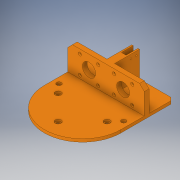
# Autodesk Inventor part: joint_1_base
Saved by Autodesk Inventor 2019 (Build 230136000, 136)
## iProperties
Created: 2019-12-25
Part Number: joint_1_base
Material: Пластик АБС
Document SubType Name: Modeling
Designer: Петров Иван
Density: 1.06 g/cm^3
Appearance: Оранжевый
Author: Петров Иван
Autodesk Inventor part; units mm, degrees
ref_plane "YZ Plane" through (0, 0, 0) normal (1, 0, 0) x (0, 1, 0)
ref_plane "XZ Plane" through (0, 0, 0) normal (0, 1, 0) x (-1, 0, 0)
ref_plane "XY Plane" through (0, 0, 0) normal (0, 0, 1) x (1, 0, 0)
sketch "Эскиз1" plane through (0, 0, 0) normal (0, 1, 0) x (-1, 0, 0)
  circle A0 centre (0, 41.5934) radius 3
  circle A1 centre (41.5934, 0) radius 3
  circle A2 centre (0, -41.5934) radius 3
  arc A3 (-20.609, 31.365) -> (-31.365, 20.609) centre (0, 0) ccw
  arc A4 (-45.7097, 6.2695) -> (-31.365, 20.609) centre (-73.1517, 48.0658) ccw
  arc A5 (-45.7097, 6.2695) -> (-45.7097, -6.2695) centre (-41.5934, 0) ccw
  arc A6 (-31.365, -20.609) -> (-45.7097, -6.2695) centre (-73.1517, -48.0658) ccw
  arc A7 (-31.365, -20.609) -> (-20.609, -31.365) centre (0, 0) ccw
  arc A8 (-6.2695, -45.7097) -> (-20.609, -31.365) centre (-48.0658, -73.1517) ccw
  arc A9 (-6.2695, -45.7097) -> (6.2695, -45.7097) centre (0, -41.5934) ccw
  arc A10 (20.609, -31.365) -> (6.2695, -45.7097) centre (48.0658, -73.1517) ccw
  arc A11 (20.609, -31.365) -> (31.365, -20.609) centre (0, 0) ccw
  arc A12 (45.7097, -6.2695) -> (31.365, -20.609) centre (73.1517, -48.0658) ccw
  arc A13 (45.7097, -6.2695) -> (45.7097, 6.2695) centre (41.5934, 0) ccw
  arc A14 (31.365, 20.609) -> (45.7097, 6.2695) centre (73.1517, 48.0658) ccw
  arc A15 (31.365, 20.609) -> (20.609, 31.365) centre (0, 0) ccw
  arc A16 (6.2695, 45.7097) -> (20.609, 31.365) centre (48.0658, 73.1517) ccw
  arc A17 (6.2695, 45.7097) -> (-6.2695, 45.7097) centre (0, 41.5934) ccw
  arc A18 (-20.609, 31.365) -> (-6.2695, 45.7097) centre (-48.0658, 73.1517) ccw
  circle A19 centre (-41.5934, 0) radius 3
  circle A20 centre (41.5934, 0) radius 3
  circle A21 centre (0, 41.5934) radius 3
  circle A22 centre (-41.5934, 0) radius 3
  circle A23 centre (0, -41.5934) radius 3
  circle A24 centre (0, 0) radius 65
  constraints: 32 point on circle, 25 centre point
extrude "Выдавливание1" add sketch "Эскиз1" along normal blind 5 contours A18 A17 A16 A15 A14 A13 A12 A11 A10 A9 A8 A7 A6 A5 A4 A3 | A24
sketch "Эскиз2" plane through (0, 5, 0) normal (0, 1, 0) x (1, 0, 0)
  circle A0 centre (0, 0) radius 65 projected
  line L0 (65, 0) -> (65, 90)
  line L1 (65, 90) -> (-65, 90)
  line L2 (-65, 90) -> (-65, 0)
  circle A1 centre (41.5934, 0) radius 3 projected
  circle A2 centre (41.5934, 0) radius 3
  circle A3 centre (-41.5934, 0) radius 3 projected
  circle A4 centre (-41.5934, 0) radius 3
  line L3 (-65, 0) -> (-44.5934, 0)
  line L4 (-38.5934, 0) -> (38.5934, 0)
  line L5 (44.5934, 0) -> (65, 0)
  dimension "d2" = 90
  constraints: 12 end point, 4 parallel, 4 point on circle, 3 horizontal, 3 perpendicular, 2 centre point, 2 coincident, 1 concentric, 1 horizontal alignment, 1 other
  measures "d2" distance of L0.end L0.start
extrude "Выдавливание2" add sketch "Эскиз2" against normal blind 5 contours L5 A1 L4 A3 L3 A0 | A0 L2 L1 L0 picked at (0, 22.5961)
chamfer "Фаска1" distance 5 angle 45 2 edges at (65, 2.5, -90) (-65, 2.5, -90)
sketch "Эскиз3" plane through (0, 5, 0) normal (0, 1, 0) x (1, 0, 0)
  line L0 (60, 90) -> (-60, 90)
  line L1 (-8, 80.5) -> (-8, 90)
  line L2 (-40, 47.8) -> (-18, 47.8)
  line L3 (-50, 49.8) -> (-50, 57.5)
  line L4 (-50, 80.5) -> (-50, 90)
  line L5 (-8, 49.8) -> (-8, 57.5)
  line L6 (8, 49.8) -> (8, 57.5)
  line L7 (8, 80.5) -> (8, 90)
  line L8 (50, 49.8) -> (50, 57.5)
  line L9 (50, 80.5) -> (50, 90)
  line L10 (18, 47.8) -> (40, 47.8)
  line L11 (-8, 47.8) -> (-50, 47.8)
  line L12 (-50, 47.8) -> (-50, 90)
  line L13 (-50, 90) -> (-8, 90)
  line L14 (-8, 90) -> (-8, 47.8)
  line L15 (8, 90) -> (50, 90)
  line L16 (50, 90) -> (50, 47.8)
  line L17 (50, 47.8) -> (8, 47.8)
  line L18 (8, 47.8) -> (8, 90)
  line L19 (-65, 0) -> (-65, 85) projected
  line L20 (65, 85) -> (65, 0) projected
  line L21 (-65, 47.8) -> (65, 47.8)
  line L22 (65, 47.8) -> (65, 39.8)
  line L23 (65, 39.8) -> (-65, 39.8)
  line L24 (-65, 39.8) -> (-65, 47.8)
  point P0 (0, 0)
  dimension "d8" = 8
  constraints: 46 end point, 6 parallel, 3 horizontal, 3 perpendicular, 3 point on line
  measures "d8" distance of L21.end L22.end
extrude "Выдавливание3" add sketch "Эскиз3" against normal blind 49 contours L21 L20 L23 L19 L11 L2 L17 L10
sketch "Эскиз5" plane through (-65, 0, -39.8) normal (0, 0, 1) x (1, 0, 0)
  circle A0 centre (94, -21) radius 11.3
  circle A1 centre (36, -21) radius 11
  line L0 (130, 0) -> (130, -44)
  line L1 (130, -44) -> (0, -44)
  point P0 (65, 0)
  dimension "d15" = 22.6
  constraints: 4 end point, 2 centre point
  measures "d15" diameter of A0
extrude "Выдавливание4" cut sketch "Эскиз5" against normal blind 44
sketch "Эскиз6" plane through (-65, 0, -39.8) normal (0, 0, 1) x (1, 0, 0)
  line L0 (111.5, -42) -> (115, -38.5)
  line L1 (115, -38.5) -> (115, -3.5)
  line L2 (115, -3.5) -> (111.5, 0)
  line L3 (111.5, 0) -> (76.5, 0)
  line L4 (76.5, 0) -> (73, -3.5)
  line L5 (73, -3.5) -> (73, -38.5)
  line L6 (73, -38.5) -> (76.5, -42)
  line L7 (76.5, -42) -> (111.5, -42)
  circle A0 centre (94, -21) radius 11.3
  circle A1 centre (109.5, -5.5) radius 1.25
  circle A2 centre (78.5, -5.5) radius 1.25
  circle A3 centre (78.5, -36.5) radius 1.25
  circle A4 centre (109.5, -36.5) radius 1.25
  line L8 (86, -48) -> (88, -48)
  line L9 (88, -41.8) -> (88, -48)
  line L10 (80.5828, -41.8) -> (88, -41.8)
  line L11 (73.2, -34.4172) -> (80.5828, -41.8)
  line L12 (73.2, -7.5828) -> (73.2, -34.4172)
  line L13 (80.5828, -0.2) -> (73.2, -7.5828)
  line L14 (107.4172, -0.2) -> (80.5828, -0.2)
  line L15 (114.8, -7.5828) -> (107.4172, -0.2)
  line L16 (114.8, -34.4172) -> (114.8, -7.5828)
  line L17 (107.4172, -41.8) -> (114.8, -34.4172)
  line L18 (100, -41.8) -> (107.4172, -41.8)
  line L19 (100, -41.8) -> (100, -48)
  line L20 (100, -48) -> (102, -48)
  line L21 (102, -48) -> (102, -42)
  line L22 (102, -42) -> (111.5, -42)
  line L23 (111.5, -42) -> (115, -38.5)
  line L24 (115, -38.5) -> (115, -3.5)
  line L25 (115, -3.5) -> (111.5, 0)
  line L26 (111.5, 0) -> (76.5, 0)
  line L27 (76.5, 0) -> (73, -3.5)
  line L28 (73, -3.5) -> (73, -38.5)
  line L29 (73, -38.5) -> (76.5, -42)
  line L30 (76.5, -42) -> (86, -42)
  line L31 (86, -42) -> (86, -48)
  circle A5 centre (94, -21) radius 11.3 projected
  circle A6 centre (36, -21) radius 11 projected
  line L32 (53.5, -42) -> (57, -38.5)
  line L33 (57, -38.5) -> (57, -3.5)
  line L34 (57, -3.5) -> (53.5, 0)
  line L35 (53.5, 0) -> (18.5, 0)
  line L36 (18.5, 0) -> (15, -3.5)
  line L37 (15, -3.5) -> (15, -38.5)
  line L38 (15, -38.5) -> (18.5, -42)
  line L39 (18.5, -42) -> (53.5, -42)
  circle A7 centre (36, -21) radius 11.3
  circle A8 centre (51.5, -5.5) radius 1.25
  circle A9 centre (20.5, -5.5) radius 1.25
  circle A10 centre (20.5, -36.5) radius 1.25
  circle A11 centre (51.5, -36.5) radius 1.25
  line L40 (28, -48) -> (30, -48)
  line L41 (30, -41.8) -> (30, -48)
  line L42 (22.5828, -41.8) -> (30, -41.8)
  line L43 (15.2, -34.4172) -> (22.5828, -41.8)
  line L44 (15.2, -7.5828) -> (15.2, -34.4172)
  line L45 (22.5828, -0.2) -> (15.2, -7.5828)
  line L46 (49.4172, -0.2) -> (22.5828, -0.2)
  line L47 (56.8, -7.5828) -> (49.4172, -0.2)
  line L48 (56.8, -34.4172) -> (56.8, -7.5828)
  line L49 (49.4172, -41.8) -> (56.8, -34.4172)
  line L50 (42, -41.8) -> (49.4172, -41.8)
  line L51 (42, -41.8) -> (42, -48)
  line L52 (42, -48) -> (44, -48)
  line L53 (44, -48) -> (44, -42)
  line L54 (44, -42) -> (53.5, -42)
  line L55 (53.5, -42) -> (57, -38.5)
  line L56 (57, -38.5) -> (57, -3.5)
  line L57 (57, -3.5) -> (53.5, 0)
  line L58 (53.5, 0) -> (18.5, 0)
  line L59 (18.5, 0) -> (15, -3.5)
  line L60 (15, -3.5) -> (15, -38.5)
  line L61 (15, -38.5) -> (18.5, -42)
  line L62 (18.5, -42) -> (28, -42)
  line L63 (28, -42) -> (28, -48)
  point P0 (65, 0)
  constraints: 128 end point, 10 centre point
extrude "Выдавливание5" cut sketch "Эскиз6" against normal blind 44 contours A1 | A2 | A3 | A4 | A8 | A9 | A10 | A11
chamfer "Фаска3" distance 8 angle 45 2 edges at (65, -44, -43.8) (-65, -44, -43.8)
sketch "Эскиз7" plane through (0, 0, 0) normal (0, -1, 0) x (1, 0, 0)
  circle A0 centre (0, 41.5934) radius 3 projected
  circle A1 centre (0, 41.5934) radius 5
  circle A2 centre (-41.5934, 0) radius 3 projected
  circle A3 centre (-41.5934, 0) radius 5
  circle A4 centre (41.5934, 0) radius 3 projected
  circle A5 centre (41.5934, 0) radius 5
  point P0 (0, 0)
  dimension "d22" = 10
  dimension "d23" = 10
  dimension "d24" = 10
  constraints: 3 centre point, 3 coincident
  measures "d22" diameter of A1
  measures "d23" diameter of A3
  measures "d24" diameter of A5
extrude "Выдавливание6" cut sketch "Эскиз7" against normal blind 3 contours A1 | A2 | A3 | A5
chamfer "Фаска4" distance 1.5 angle 45 8 edges at (43.25, -36.5, -39.8) (12.25, -36.5, -39.8) (12.25, -5.5, -39.8) (43.25, -5.5, -39.8) (-14.75, -36.5, -39.8) (-14.75, -5.5, -39.8) (-45.75, -5.5, -39.8) (-45.75, -36.5, -39.8)
sketch "Эскиз8" plane through (0, 5, 0) normal (0, 1, 0) x (1, 0, 0)
  circle A0 centre (-55, 14.8) radius 4
  circle A1 centre (55, 14.8) radius 4
  line L0 (60, 90) -> (-60, 90)
  point P0 (0, 0)
  constraints: 2 centre point, 2 end point
extrude "Выдавливание7" cut sketch "Эскиз8" against normal through all
sketch "Эскиз9" plane through (65, 0, -47.8) normal (0, 0, -1) x (-1, 0, 0)
  line L0 (122, -44) -> (8, -44) projected
  line L1 (65, -44) -> (65, -22)
  line L2 (71.5, 0) -> (58.5, 0)
  line L3 (58.5, 0) -> (58.5, -44)
  line L4 (58.5, -44) -> (71.5, -44)
  line L5 (71.5, -44) -> (71.5, 0)
  line L6 (71.5, 0) -> (58.5, -44) construction
  line L7 (58.5, 0) -> (71.5, -44) construction
  point P0 (65, 0)
  dimension "d32" = 13
  dimension "d34" = 22
  constraints: 14 end point, 3 midpoint, 2 parallel, 1 horizontal, 1 perpendicular, 1 point on line, 1 vertical
  measures "d32" distance of L4.end L3.end
  measures "d34" distance of L1.start L1.end
extrude "Выдавливание8" add sketch "Эскиз9" along normal up to surface (42.2 mm away)
sketch "Эскиз10" plane through (0, -44, 0) normal (0, -1, 0) x (1, 0, 0)
  line L0 (-6.5, -90) -> (6.5, -90) projected
  line L1 (0, -90) -> (0, -79.9)
  line L2 (-4, -90) -> (4, -90)
  line L3 (4, -90) -> (4, -69.8)
  line L4 (4, -69.8) -> (-4, -69.8)
  line L5 (-4, -69.8) -> (-4, -90)
  line L6 (-4, -90) -> (4, -69.8) construction
  line L7 (4, -90) -> (-4, -69.8) construction
  line L8 (-57, -47.8) -> (-57, -39.8) projected
  line L9 (-57, -47.8) -> (-6.5, -47.8) projected
  line L10 (-6.5, -47.8) -> (-6.5, -90) projected
  line L11 (-6.5, -90) -> (6.5, -90) projected
  line L12 (6.5, -47.8) -> (6.5, -90) projected
  line L13 (6.5, -47.8) -> (57, -47.8) projected
  line L14 (57, -39.8) -> (57, -47.8) projected
  line L15 (57, -39.8) -> (-57, -39.8) projected
  line L16 (-6.5, -47.8) -> (-6.5, -90) projected
  line L17 (-6.5, -47.8) -> (6.5, -47.8)
  line L18 (6.5, -47.8) -> (6.5, -90)
  line L19 (4, -90) -> (6.5, -90)
  line L20 (-4, -90) -> (-6.5, -90)
  line L21 (-6.5, -90) -> (-6.5, -47.8)
  point P0 (0, 0)
  dimension "d37" = 10.1
  dimension "d38" = 8
  dimension "d39" = 20.2
  constraints: 24 end point, 3 equal length, 3 midpoint, 3 perpendicular, 1 horizontal, 1 vertical
  measures "d37" distance of L1.start L1.end
  measures "d38" distance of L4.end L3.end
  measures "d39" distance of L3.end L2.end
extrude "Выдавливание9" cut sketch "Эскиз10" against normal blind 18 contours L5 L4 L3 L0
sketch "Эскиз11" plane through (-6.5, -44, -47.8) normal (-1, 0, 0) x (0, 0, 1)
  line L0 (-42.2, 18) -> (-22, 18) projected
  line L1 (-22, 0) -> (-22, 18) projected
  arc A0 (-42.133, -0.5583) -> (-42.033, -0.4583) centre (-42.133, -0.4583) ccw
  line L2 (-42.033, -0.4583) -> (-42.033, 8.6917)
  arc A1 (-42.033, 8.6917) -> (-42.133, 8.7917) centre (-42.133, 8.6917) ccw
  line L3 (-22.333, -1.0583) -> (-22.8455, -1.0583)
  line L4 (-22.8455, -1.0583) -> (-22.9372, 0.3757)
  arc A2 (-22.9372, 0.3757) -> (-27.1287, 0.3757) centre (-25.033, 0.2417) ccw
  line L5 (-27.1287, 0.3757) -> (-27.2204, -1.0583)
  line L6 (-27.2204, -1.0583) -> (-31.5087, -1.0583)
  arc A3 (-31.5794, -1.029) -> (-31.5087, -1.0583) centre (-31.5087, -0.9583) ccw
  line L7 (-31.5794, -1.029) -> (-31.9037, -0.7048)
  arc A4 (-31.9037, -0.7048) -> (-32.2572, -0.5583) centre (-32.2572, -1.0583) ccw
  line L8 (-32.2572, -0.5583) -> (-41.933, -0.5583)
  arc A5 (-42.033, -0.4583) -> (-41.933, -0.5583) centre (-41.933, -0.4583) ccw
  arc A6 (-41.933, 8.7917) -> (-42.033, 8.6917) centre (-41.933, 8.6917) ccw
  line L9 (-41.933, 8.7917) -> (-39.0072, 8.7917)
  arc A7 (-39.0072, 8.7917) -> (-38.6537, 8.9381) centre (-39.0072, 9.2917) ccw
  line L10 (-38.6537, 8.9381) -> (-38.3294, 9.2624)
  arc A8 (-38.2587, 9.2917) -> (-38.3294, 9.2624) centre (-38.2587, 9.1917) ccw
  line L11 (-38.2587, 9.2917) -> (-35.5072, 9.2917)
  arc A9 (-35.4365, 9.2624) -> (-35.5072, 9.2917) centre (-35.5072, 9.1917) ccw
  line L12 (-35.4365, 9.2624) -> (-35.1122, 8.9381)
  arc A10 (-35.1122, 8.9381) -> (-34.7587, 8.7917) centre (-34.7587, 9.2917) ccw
  line L13 (-34.7587, 8.7917) -> (-29.5072, 8.7917)
  arc A11 (-29.5072, 8.7917) -> (-29.1537, 8.9381) centre (-29.5072, 9.2917) ccw
  line L14 (-29.1537, 8.9381) -> (-28.8294, 9.2624)
  arc A12 (-28.7587, 9.2917) -> (-28.8294, 9.2624) centre (-28.7587, 9.1917) ccw
  line L15 (-28.7587, 9.2917) -> (-26.0072, 9.2917)
  arc A13 (-25.9365, 9.2624) -> (-26.0072, 9.2917) centre (-26.0072, 9.1917) ccw
  line L16 (-25.9365, 9.2624) -> (-25.6122, 8.9381)
  arc A14 (-25.6122, 8.9381) -> (-25.2587, 8.7917) centre (-25.2587, 9.2917) ccw
  line L17 (-25.2587, 8.7917) -> (-22.333, 8.7917)
  arc A15 (-22.233, 8.6917) -> (-22.333, 8.7917) centre (-22.333, 8.6917) ccw
  line L18 (-22.233, 8.6917) -> (-22.233, -0.9583)
  arc A16 (-22.333, -1.0583) -> (-22.233, -0.9583) centre (-22.333, -0.9583) ccw
  circle A17 centre (-27.383, 6.7417) radius 1.25
  circle A18 centre (-36.883, 6.7417) radius 1.25
  line L19 (-38.0563, 4.4917) -> (-37.4396, 3.1917)
  line L20 (-37.4396, 3.1917) -> (-37.423, 3.1917)
  line L21 (-37.423, 3.1917) -> (-36.823, 4.4917)
  line L22 (-36.823, 4.4917) -> (-36.9498, 4.4917)
  line L23 (-36.9498, 4.4917) -> (-37.142, 4.075)
  line L24 (-37.142, 4.075) -> (-37.7313, 4.075)
  line L25 (-37.7313, 4.075) -> (-37.9289, 4.4917)
  line L26 (-37.9289, 4.4917) -> (-38.0563, 4.4917)
  spline S0 degree 3 poles (-35.2363, 3.5552) (-35.2365, 3.5463) (-35.237, 3.5289) (-35.2411, 3.5032) (-35.2473, 3.4785) (-35.2562, 3.4546) (-35.2679, 3.4318) (-35.2822, 3.41) (-35.2987, 3.389) (-35.3178, 3.3692) (-35.3387, 3.3511) (-35.3609, 3.3351) (-35.3843, 3.3217) (-35.4089, 3.3108) (-35.4346, 3.3022) (-35.4615, 3.2962) (-35.4895, 3.2924) (-35.5086, 3.2919) (-35.5183, 3.2917) knots 0 0 0 0 0.061965 0.122122 0.180988 0.239933 0.299906 0.359989 0.421776 0.486576 0.551535 0.615018 0.677259 0.73973 0.80305 0.866495 0.931973 1 1 1 1
  spline S1 degree 3 poles (-35.5183, 3.2917) (-35.5285, 3.2919) (-35.5485, 3.2925) (-35.5778, 3.2961) (-35.6057, 3.3024) (-35.6324, 3.311) (-35.6579, 3.322) (-35.682, 3.3356) (-35.7046, 3.3518) (-35.7259, 3.3703) (-35.7456, 3.3908) (-35.7628, 3.4137) (-35.7779, 3.4385) (-35.7911, 3.4652) (-35.8017, 3.494) (-35.8099, 3.5248) (-35.8164, 3.5575) (-35.8185, 3.5801) (-35.8196, 3.5917) knots 0 0 0 0 0.064439 0.126547 0.186887 0.245878 0.304041 0.362191 0.420976 0.48066 0.5406 0.600689 0.661936 0.724443 0.789038 0.856314 0.926352 1 1 1 1
  line L27 (-35.8196, 3.5917) -> (-35.9363, 3.5917)
  spline S2 degree 3 poles (-35.9363, 3.5917) (-35.9355, 3.5762) (-35.934, 3.5458) (-35.927, 3.5015) (-35.917, 3.4591) (-35.9029, 3.4191) (-35.8853, 3.3809) (-35.8642, 3.3449) (-35.8393, 3.3111) (-35.811, 3.2799) (-35.7802, 3.2512) (-35.7471, 3.2264) (-35.7122, 3.2055) (-35.6758, 3.188) (-35.6373, 3.1749) (-35.5973, 3.1652) (-35.5554, 3.1593) (-35.5268, 3.1587) (-35.5123, 3.1583) knots 0 0 0 0 0.068791 0.135103 0.198979 0.261904 0.323495 0.385195 0.446969 0.509765 0.572251 0.633405 0.693251 0.752583 0.812579 0.873275 0.93555 1 1 1 1
  spline S3 degree 3 poles (-35.5123, 3.1583) (-35.4981, 3.1587) (-35.4701, 3.1593) (-35.4292, 3.165) (-35.3903, 3.1738) (-35.3534, 3.1862) (-35.3188, 3.2028) (-35.2864, 3.2228) (-35.2556, 3.2459) (-35.2279, 3.2731) (-35.2024, 3.3021) (-35.1805, 3.3331) (-35.1617, 3.3652) (-35.146, 3.3985) (-35.1345, 3.4333) (-35.1257, 3.4693) (-35.1208, 3.5066) (-35.12, 3.5319) (-35.1196, 3.5448) knots 0 0 0 0 0.069475 0.136517 0.200789 0.26383 0.325735 0.387291 0.449509 0.512968 0.576275 0.63758 0.697903 0.757172 0.816599 0.876653 0.93729 1 1 1 1
  spline S4 degree 3 poles (-35.1196, 3.5448) (-35.1203, 3.5629) (-35.1215, 3.5988) (-35.1322, 3.6516) (-35.1488, 3.7027) (-35.1689, 3.7438) (-35.1891, 3.7769) (-35.2073, 3.8042) (-35.2287, 3.8336) (-35.2535, 3.865) (-35.2811, 3.8986) (-35.312, 3.9344) (-35.3462, 3.9721) (-35.3702, 3.9979) (-35.3826, 4.0112) knots 0 0 0 0 0.098702 0.195672 0.292422 0.391343 0.444462 0.504229 0.570352 0.642546 0.722288 0.807921 0.90047 1 1 1 1
  line L28 (-35.3826, 4.0112) -> (-35.7079, 4.3583)
  line L29 (-35.7079, 4.3583) -> (-35.103, 4.3583)
  line L30 (-35.103, 4.3583) -> (-35.103, 4.4917)
  line L31 (-35.103, 4.4917) -> (-35.9863, 4.4917)
  line L32 (-35.9863, 4.4917) -> (-35.4821, 3.9537)
  spline S5 degree 3 poles (-35.4821, 3.9537) (-35.4699, 3.9408) (-35.4463, 3.9162) (-35.4129, 3.8803) (-35.383, 3.847) (-35.3562, 3.8163) (-35.3333, 3.7878) (-35.3129, 3.7625) (-35.2965, 3.7392) (-35.2788, 3.7122) (-35.2617, 3.6792) (-35.2469, 3.6389) (-35.2379, 3.5974) (-35.2368, 3.5693) (-35.2363, 3.5552) knots 0 0 0 0 0.110803 0.212829 0.306101 0.390647 0.466924 0.534481 0.593587 0.644557 0.7362 0.825024 0.911986 1 1 1 1
  line L33 (-34.7263, 3.8417) -> (-34.593, 3.1917)
  line L34 (-34.593, 3.1917) -> (-34.0596, 3.1917)
  line L35 (-34.0596, 3.1917) -> (-34.0596, 3.325)
  line L36 (-34.0596, 3.325) -> (-34.5018, 3.325)
  line L37 (-34.5018, 3.325) -> (-34.5719, 3.6669)
  spline S6 degree 3 poles (-34.5719, 3.6669) (-34.5581, 3.6631) (-34.5314, 3.6558) (-34.4921, 3.6476) (-34.4547, 3.6427) (-34.4305, 3.642) (-34.4187, 3.6417) knots 0 0 0 0 0.275068 0.532901 0.773973 1 1 1 1
  spline S7 degree 3 poles (-34.4187, 3.6417) (-34.4042, 3.642) (-34.3757, 3.6426) (-34.3339, 3.6485) (-34.294, 3.6579) (-34.2562, 3.6709) (-34.2202, 3.6876) (-34.1865, 3.7084) (-34.1544, 3.7328) (-34.1248, 3.7608) (-34.0978, 3.7916) (-34.0741, 3.8247) (-34.054, 3.8598) (-34.0378, 3.8972) (-34.0249, 3.9366) (-34.0163, 3.9783) (-34.0106, 4.0219) (-34.01, 4.0517) (-34.0096, 4.0669) knots 0 0 0 0 0.065808 0.129394 0.190894 0.251281 0.310815 0.370371 0.430768 0.492881 0.555104 0.616067 0.677256 0.73826 0.800762 0.864778 0.931045 1 1 1 1
  spline S8 degree 3 poles (-34.0096, 4.0669) (-34.0099, 4.0775) (-34.0104, 4.0986) (-34.0129, 4.1298) (-34.0177, 4.1604) (-34.0241, 4.1904) (-34.0325, 4.2196) (-34.0426, 4.2482) (-34.055, 4.2759) (-34.0686, 4.3032) (-34.084, 4.3293) (-34.101, 4.3536) (-34.1189, 4.3767) (-34.1383, 4.3982) (-34.1591, 4.418) (-34.1813, 4.4361) (-34.2046, 4.453) (-34.2293, 4.468) (-34.255, 4.4817) (-34.282, 4.4929) (-34.3096, 4.503) (-34.3384, 4.511) (-34.3681, 4.5173) (-34.3989, 4.5216) (-34.4307, 4.5247) (-34.4522, 4.5249) (-34.463, 4.525) knots 0 0 0 0 0.044014 0.087434 0.130118 0.172554 0.214555 0.256298 0.298438 0.340849 0.382715 0.423924 0.464246 0.504074 0.543862 0.583567 0.623094 0.663229 0.703551 0.743938 0.784541 0.82575 0.867757 0.910745 0.954914 1 1 1 1
  spline S9 degree 3 poles (-34.463, 4.525) (-34.476, 4.5248) (-34.5014, 4.5242) (-34.5388, 4.519) (-34.5747, 4.5114) (-34.6089, 4.5) (-34.6418, 4.4858) (-34.6727, 4.4677) (-34.7027, 4.4473) (-34.7304, 4.4232) (-34.756, 4.3969) (-34.779, 4.3683) (-34.7995, 4.3379) (-34.8171, 4.3057) (-34.8322, 4.2716) (-34.844, 4.2355) (-34.8535, 4.1976) (-34.8576, 4.1716) (-34.8596, 4.1583) knots 0 0 0 0 0.065421 0.128708 0.190236 0.250724 0.310637 0.370766 0.431615 0.493523 0.555883 0.617342 0.678668 0.740711 0.802985 0.866803 0.932347 1 1 1 1
  line L38 (-34.8596, 4.1583) -> (-34.743, 4.1583)
  spline S10 degree 3 poles (-34.743, 4.1583) (-34.7401, 4.1707) (-34.7346, 4.1946) (-34.7225, 4.228) (-34.7077, 4.2579) (-34.69, 4.2845) (-34.669, 4.3076) (-34.6451, 4.3283) (-34.6182, 4.3469) (-34.5883, 4.3625) (-34.5568, 4.3757) (-34.5239, 4.3845) (-34.4903, 4.3907) (-34.4676, 4.3914) (-34.4562, 4.3917) knots 0 0 0 0 0.094687 0.181994 0.264377 0.34218 0.418618 0.496509 0.577369 0.661511 0.746733 0.831258 0.915206 1 1 1 1
  spline S11 degree 3 poles (-34.4562, 4.3917) (-34.4451, 4.3914) (-34.4232, 4.3908) (-34.391, 4.3862) (-34.3598, 4.379) (-34.3301, 4.3684) (-34.3013, 4.3554) (-34.2741, 4.3388) (-34.2478, 4.3197) (-34.2231, 4.2978) (-34.2005, 4.2737) (-34.1806, 4.2479) (-34.1639, 4.2204) (-34.1499, 4.1916) (-34.1393, 4.1612) (-34.1317, 4.1295) (-34.1272, 4.0962) (-34.1266, 4.0735) (-34.1263, 4.062) knots 0 0 0 0 0.064207 0.126425 0.18768 0.248216 0.308305 0.369661 0.431699 0.495947 0.559758 0.622295 0.683911 0.745092 0.80674 0.869087 0.93329 1 1 1 1
  spline S12 degree 3 poles (-34.1263, 4.062) (-34.1265, 4.0516) (-34.127, 4.0311) (-34.1309, 4.0013) (-34.1377, 3.973) (-34.1472, 3.9462) (-34.1592, 3.9209) (-34.1738, 3.897) (-34.1914, 3.8748) (-34.2115, 3.8543) (-34.2335, 3.8354) (-34.2578, 3.8193) (-34.2839, 3.8058) (-34.3115, 3.7941) (-34.3412, 3.7857) (-34.3724, 3.7794) (-34.4055, 3.7758) (-34.4282, 3.7753) (-34.4398, 3.775) knots 0 0 0 0 0.065351 0.127916 0.18836 0.247216 0.30563 0.36377 0.422661 0.482687 0.5433 0.604118 0.664965 0.727413 0.791468 0.858055 0.927037 1 1 1 1
  spline S13 degree 3 poles (-34.4398, 3.775) (-34.4499, 3.7752) (-34.4707, 3.7757) (-34.5026, 3.7789) (-34.5362, 3.7842) (-34.5712, 3.7915) (-34.6078, 3.801) (-34.646, 3.8124) (-34.6857, 3.8261) (-34.7125, 3.8364) (-34.7263, 3.8417) knots 0 0 0 0 0.102203 0.211023 0.3251 0.446502 0.573788 0.708901 0.850358 1 1 1 1
  line L39 (-31.2796, 4.4917) -> (-30.663, 3.1917)
  line L40 (-30.663, 3.1917) -> (-30.6463, 3.1917)
  line L41 (-30.6463, 3.1917) -> (-30.0463, 4.4917)
  line L42 (-30.0463, 4.4917) -> (-30.1731, 4.4917)
  line L43 (-30.1731, 4.4917) -> (-30.3653, 4.075)
  line L44 (-30.3653, 4.075) -> (-30.9546, 4.075)
  line L45 (-30.9546, 4.075) -> (-31.1523, 4.4917)
  line L46 (-31.1523, 4.4917) -> (-31.2796, 4.4917)
  spline S14 degree 3 poles (-29.7696, 3.8341) (-29.769, 3.8107) (-29.7679, 3.7647) (-29.7583, 3.6972) (-29.7427, 3.6325) (-29.7207, 3.5708) (-29.6927, 3.5117) (-29.6581, 3.4557) (-29.6174, 3.4024) (-29.5708, 3.3526) (-29.5197, 3.3071) (-29.465, 3.267) (-29.4068, 3.2337) (-29.3457, 3.2058) (-29.2812, 3.1844) (-29.2136, 3.1695) (-29.1429, 3.1601) (-29.0947, 3.1589) (-29.0701, 3.1583) knots 0 0 0 0 0.064558 0.127014 0.187955 0.248014 0.307748 0.368235 0.42947 0.492743 0.556258 0.618217 0.679655 0.741246 0.803415 0.866815 0.932328 1 1 1 1
  spline S15 degree 3 poles (-29.0701, 3.1583) (-29.0552, 3.1585) (-29.0256, 3.1589) (-28.9819, 3.1623) (-28.9393, 3.1681) (-28.8979, 3.1759) (-28.8573, 3.1857) (-28.818, 3.1984) (-28.7797, 3.2129) (-28.7427, 3.2296) (-28.7071, 3.2483) (-28.6729, 3.2689) (-28.6404, 3.2913) (-28.6094, 3.3153) (-28.5804, 3.3414) (-28.5525, 3.369) (-28.5268, 3.3988) (-28.5109, 3.4197) (-28.503, 3.4302) knots 0 0 0 0 0.068548 0.135683 0.201215 0.265682 0.329267 0.392395 0.45507 0.517127 0.57879 0.63974 0.700192 0.759806 0.819628 0.879355 0.939512 1 1 1 1
  line L47 (-28.503, 3.4302) -> (-28.605, 3.5083)
  spline S16 degree 3 poles (-28.605, 3.5083) (-28.6123, 3.4997) (-28.6268, 3.4824) (-28.6501, 3.4582) (-28.6743, 3.4355) (-28.6995, 3.4143) (-28.7262, 3.3952) (-28.7536, 3.3772) (-28.7823, 3.3612) (-28.822, 3.3417) (-28.8738, 3.3214) (-28.9391, 3.3043) (-29.0073, 3.2934) (-29.0538, 3.2923) (-29.0774, 3.2917) knots 0 0 0 0 0.063163 0.125475 0.187121 0.248294 0.309295 0.36985 0.430973 0.492456 0.616148 0.740844 0.868183 1 1 1 1
  spline S17 degree 3 poles (-29.0774, 3.2917) (-29.0905, 3.2918) (-29.1164, 3.2921) (-29.1549, 3.2961) (-29.1927, 3.3016) (-29.2297, 3.3098) (-29.266, 3.3202) (-29.3017, 3.3326) (-29.3363, 3.348) (-29.3703, 3.365) (-29.4029, 3.3841) (-29.4338, 3.4051) (-29.4627, 3.4275) (-29.4899, 3.4515) (-29.5152, 3.477) (-29.5385, 3.5042) (-29.5598, 3.5332) (-29.5793, 3.5634) (-29.5969, 3.5948) (-29.6116, 3.6275) (-29.6246, 3.6609) (-29.6349, 3.6955) (-29.643, 3.731) (-29.6486, 3.7675) (-29.6525, 3.8049) (-29.6528, 3.8302) (-29.653, 3.843) knots 0 0 0 0 0.043955 0.087502 0.130463 0.172752 0.215403 0.25765 0.300153 0.343121 0.385925 0.427686 0.468818 0.509492 0.549883 0.58998 0.630405 0.670869 0.711384 0.751627 0.791776 0.832459 0.873319 0.914543 0.956924 1 1 1 1
  spline S18 degree 3 poles (-29.653, 3.843) (-29.6525, 3.8622) (-29.6516, 3.8999) (-29.6434, 3.9552) (-29.6309, 4.0081) (-29.6123, 4.0584) (-29.5893, 4.1066) (-29.5602, 4.1521) (-29.5266, 4.1953) (-29.4878, 4.2353) (-29.4453, 4.2719) (-29.3998, 4.3042) (-29.3512, 4.331) (-29.3001, 4.3534) (-29.2463, 4.3706) (-29.1897, 4.3826) (-29.1304, 4.3905) (-29.09, 4.3913) (-29.0694, 4.3917) knots 0 0 0 0 0.064323 0.12629 0.186726 0.246146 0.305576 0.365429 0.426326 0.48884 0.551725 0.613919 0.675484 0.737334 0.800229 0.864502 0.931041 1 1 1 1
  spline S19 degree 3 poles (-29.0694, 4.3917) (-29.0467, 4.391) (-29.002, 4.3898) (-28.9365, 4.3794) (-28.8738, 4.3624) (-28.8139, 4.3387) (-28.7569, 4.3078) (-28.7028, 4.2704) (-28.6516, 4.2261) (-28.6208, 4.1923) (-28.605, 4.175) knots 0 0 0 0 0.128515 0.252949 0.374755 0.49594 0.617181 0.740909 0.867811 1 1 1 1
  line L48 (-28.605, 4.175) -> (-28.503, 4.2524)
  spline S20 degree 3 poles (-28.503, 4.2524) (-28.5112, 4.263) (-28.5276, 4.2841) (-28.5541, 4.3139) (-28.5821, 4.342) (-28.6117, 4.368) (-28.6425, 4.3926) (-28.6752, 4.415) (-28.7094, 4.4355) (-28.7448, 4.4543) (-28.7815, 4.471) (-28.8193, 4.4853) (-28.8583, 4.4976) (-28.8983, 4.5077) (-28.9394, 4.5156) (-28.9815, 4.5209) (-29.0247, 4.5245) (-29.0538, 4.5248) (-29.0686, 4.525) knots 0 0 0 0 0.061674 0.123053 0.183475 0.243727 0.304279 0.364863 0.425946 0.487391 0.54922 0.611144 0.673529 0.736961 0.800785 0.866013 0.932101 1 1 1 1
  spline S21 degree 3 poles (-29.0686, 4.525) (-29.0826, 4.5249) (-29.1102, 4.5247) (-29.151, 4.5216) (-29.1908, 4.5173) (-29.2293, 4.5109) (-29.2669, 4.5034) (-29.3031, 4.4933) (-29.3384, 4.4819) (-29.3725, 4.4686) (-29.4056, 4.4535) (-29.4375, 4.4365) (-29.4682, 4.4177) (-29.498, 4.3975) (-29.5264, 4.3752) (-29.5538, 4.3512) (-29.5802, 4.3255) (-29.5966, 4.307) (-29.6048, 4.2977) knots 0 0 0 0 0.069663 0.13775 0.203917 0.26878 0.332414 0.394754 0.45618 0.516996 0.577396 0.637198 0.696999 0.756756 0.816554 0.876948 0.938132 1 1 1 1
  spline S22 degree 3 poles (-29.6048, 4.2977) (-29.6179, 4.2815) (-29.6441, 4.2493) (-29.6776, 4.1972) (-29.7062, 4.1428) (-29.7294, 4.0859) (-29.7475, 4.0264) (-29.7601, 3.9645) (-29.7682, 3.9001) (-29.7692, 3.8564) (-29.7696, 3.8341) knots 0 0 0 0 0.124329 0.247156 0.36878 0.490734 0.613614 0.738958 0.867311 1 1 1 1
  line L49 (-26.697, 3.2417) -> (-26.9098, 3.2417)
  line L50 (-27.0973, 4.3417) -> (-26.697, 3.2417)
  line L51 (-26.5973, 4.3417) -> (-27.0973, 4.3417)
  line L52 (-26.197, 3.2417) -> (-26.5973, 4.3417)
  line L53 (-25.9841, 3.2417) -> (-26.197, 3.2417)
  line L54 (-26.3845, 4.3417) -> (-25.9841, 3.2417)
  line L55 (-26.1845, 4.3417) -> (-26.3845, 4.3417)
  line L56 (-26.2573, 4.5417) -> (-26.1845, 4.3417)
  line L57 (-27.383, 4.5417) -> (-26.2573, 4.5417)
  line L58 (-26.9098, 3.2417) -> (-27.383, 4.5417)
  line L59 (-32.073, 4.4917) -> (-32.0896, 4.4917)
  line L60 (-32.0896, 4.4917) -> (-32.6396, 3.1917)
  line L61 (-32.6396, 3.1917) -> (-32.5146, 3.1917)
  line L62 (-32.5146, 3.1917) -> (-32.0813, 4.2162)
  line L63 (-32.0813, 4.2162) -> (-31.648, 3.1917)
  line L64 (-31.648, 3.1917) -> (-31.523, 3.1917)
  line L65 (-31.523, 3.1917) -> (-32.073, 4.4917)
  spline S23 degree 3 poles (-32.883, 3.8422) (-32.8832, 3.8621) (-32.8837, 3.9008) (-32.8861, 3.9575) (-32.8909, 4.011) (-32.8969, 4.0614) (-32.9053, 4.1086) (-32.9155, 4.1527) (-32.9269, 4.1939) (-32.941, 4.2319) (-32.9564, 4.2671) (-32.9731, 4.3001) (-32.991, 4.331) (-33.0106, 4.3596) (-33.0314, 4.3861) (-33.0539, 4.41) (-33.0776, 4.432) (-33.1026, 4.4516) (-33.1288, 4.4687) (-33.1555, 4.484) (-33.1833, 4.4963) (-33.2115, 4.5069) (-33.2405, 4.515) (-33.2703, 4.5206) (-33.3007, 4.5246) (-33.3213, 4.5249) (-33.3317, 4.525) knots 0 0 0 0 0.065063 0.126773 0.185516 0.240765 0.29298 0.34225 0.388919 0.432776 0.474628 0.514775 0.553606 0.591426 0.628028 0.663804 0.698984 0.733591 0.767628 0.801208 0.834264 0.866981 0.89972 0.932702 0.966176 1 1 1 1
  spline S24 degree 3 poles (-33.3317, 4.525) (-33.3419, 4.5248) (-33.3621, 4.5245) (-33.3921, 4.521) (-33.4212, 4.5153) (-33.4495, 4.5073) (-33.4772, 4.4976) (-33.504, 4.4849) (-33.5301, 4.4703) (-33.5555, 4.4537) (-33.5796, 4.4346) (-33.6027, 4.4135) (-33.6241, 4.3899) (-33.644, 4.3641) (-33.663, 4.3363) (-33.6804, 4.3063) (-33.6965, 4.274) (-33.7112, 4.2394) (-33.7243, 4.2018) (-33.7358, 4.1609) (-33.7449, 4.1163) (-33.7527, 4.0683) (-33.759, 4.0168) (-33.7633, 3.9617) (-33.7659, 3.9031) (-33.7662, 3.8629) (-33.7663, 3.8422) knots 0 0 0 0 0.033787 0.066622 0.099285 0.131361 0.163585 0.196104 0.228902 0.262158 0.295991 0.330218 0.36506 0.400951 0.43762 0.475708 0.515381 0.556414 0.599765 0.646424 0.696431 0.749782 0.806573 0.867436 0.931887 1 1 1 1
  spline S25 degree 3 poles (-33.7663, 3.8422) (-33.7662, 3.8214) (-33.7659, 3.7809) (-33.7633, 3.7219) (-33.7589, 3.6666) (-33.7529, 3.6149) (-33.7456, 3.5669) (-33.7359, 3.5226) (-33.7248, 3.4818) (-33.712, 3.4445) (-33.6975, 3.4101) (-33.6818, 3.378) (-33.6641, 3.3483) (-33.6455, 3.3204) (-33.6253, 3.2948) (-33.604, 3.2711) (-33.5808, 3.25) (-33.5565, 3.2307) (-33.5309, 3.2139) (-33.5047, 3.199) (-33.4776, 3.1863) (-33.4498, 3.1763) (-33.4213, 3.168) (-33.3921, 3.1624) (-33.3621, 3.1589) (-33.3419, 3.1585) (-33.3317, 3.1583) knots 0 0 0 0 0.068595 0.133246 0.194313 0.251279 0.304513 0.354235 0.400481 0.443411 0.484015 0.523252 0.561042 0.5979 0.633518 0.668314 0.702496 0.736685 0.770293 0.803437 0.835913 0.86846 0.900847 0.933467 0.966258 1 1 1 1
  spline S26 degree 3 poles (-33.3317, 3.1583) (-33.3213, 3.1585) (-33.3008, 3.1589) (-33.2704, 3.1623) (-33.2407, 3.1681) (-33.2118, 3.1762) (-33.1835, 3.1863) (-33.1561, 3.199) (-33.1292, 3.2137) (-33.1035, 3.2311) (-33.0785, 3.2504) (-33.055, 3.2722) (-33.0328, 3.2963) (-33.0117, 3.3225) (-32.9924, 3.3512) (-32.974, 3.3819) (-32.9575, 3.4153) (-32.9416, 3.4506) (-32.9279, 3.489) (-32.9156, 3.5301) (-32.9056, 3.5745) (-32.8973, 3.622) (-32.8908, 3.6726) (-32.8861, 3.7264) (-32.8837, 3.7833) (-32.8832, 3.8222) (-32.883, 3.8422) knots 0 0 0 0 0.033788 0.067194 0.099862 0.132567 0.165151 0.197913 0.231319 0.265083 0.299255 0.334399 0.369943 0.406284 0.444064 0.482998 0.523354 0.565537 0.609613 0.656391 0.705885 0.758325 0.813832 0.872795 0.934722 1 1 1 1
  line L66 (-39.033, 3.8417) -> (-38.8996, 3.1917)
  line L67 (-38.8996, 3.1917) -> (-38.3663, 3.1917)
  line L68 (-38.3663, 3.1917) -> (-38.3663, 3.325)
  line L69 (-38.3663, 3.325) -> (-38.8085, 3.325)
  line L70 (-38.8085, 3.325) -> (-38.8785, 3.6669)
  spline S27 degree 3 poles (-38.8785, 3.6669) (-38.8648, 3.6631) (-38.8381, 3.6558) (-38.7987, 3.6476) (-38.7614, 3.6427) (-38.7371, 3.642) (-38.7254, 3.6417) knots 0 0 0 0 0.275068 0.532901 0.773973 1 1 1 1
  spline S28 degree 3 poles (-38.7254, 3.6417) (-38.7109, 3.642) (-38.6823, 3.6426) (-38.6406, 3.6485) (-38.6007, 3.6579) (-38.5628, 3.6709) (-38.5269, 3.6876) (-38.4931, 3.7084) (-38.4611, 3.7328) (-38.4314, 3.7608) (-38.4045, 3.7916) (-38.3808, 3.8247) (-38.3607, 3.8598) (-38.3445, 3.8972) (-38.3316, 3.9366) (-38.323, 3.9783) (-38.3173, 4.0219) (-38.3166, 4.0517) (-38.3163, 4.0669) knots 0 0 0 0 0.065808 0.129394 0.190894 0.251281 0.310815 0.370371 0.430768 0.492881 0.555104 0.616067 0.677256 0.73826 0.800762 0.864778 0.931045 1 1 1 1
  spline S29 degree 3 poles (-38.3163, 4.0669) (-38.3165, 4.0775) (-38.317, 4.0986) (-38.3195, 4.1298) (-38.3243, 4.1604) (-38.3308, 4.1904) (-38.3392, 4.2196) (-38.3493, 4.2482) (-38.3617, 4.2759) (-38.3753, 4.3032) (-38.3906, 4.3293) (-38.4076, 4.3536) (-38.4256, 4.3767) (-38.4449, 4.3982) (-38.4658, 4.418) (-38.488, 4.4361) (-38.5112, 4.453) (-38.536, 4.468) (-38.5617, 4.4817) (-38.5887, 4.4929) (-38.6163, 4.503) (-38.645, 4.511) (-38.6748, 4.5173) (-38.7056, 4.5216) (-38.7373, 4.5247) (-38.7588, 4.5249) (-38.7697, 4.525) knots 0 0 0 0 0.044014 0.087434 0.130118 0.172554 0.214555 0.256298 0.298438 0.340849 0.382715 0.423924 0.464246 0.504074 0.543862 0.583567 0.623094 0.663229 0.703551 0.743938 0.784541 0.82575 0.867757 0.910745 0.954914 1 1 1 1
  spline S30 degree 3 poles (-38.7697, 4.525) (-38.7826, 4.5248) (-38.8081, 4.5242) (-38.8455, 4.519) (-38.8814, 4.5114) (-38.9156, 4.5) (-38.9484, 4.4858) (-38.9794, 4.4677) (-39.0093, 4.4473) (-39.037, 4.4232) (-39.0627, 4.3969) (-39.0857, 4.3683) (-39.1062, 4.3379) (-39.1238, 4.3057) (-39.1389, 4.2716) (-39.1507, 4.2355) (-39.1602, 4.1976) (-39.1642, 4.1716) (-39.1663, 4.1583) knots 0 0 0 0 0.065421 0.128708 0.190236 0.250724 0.310637 0.370766 0.431615 0.493523 0.555883 0.617342 0.678668 0.740711 0.802985 0.866803 0.932347 1 1 1 1
  line L71 (-39.1663, 4.1583) -> (-39.0496, 4.1583)
  spline S31 degree 3 poles (-39.0496, 4.1583) (-39.0468, 4.1707) (-39.0412, 4.1946) (-39.0291, 4.228) (-39.0143, 4.2579) (-38.9967, 4.2845) (-38.9757, 4.3076) (-38.9517, 4.3283) (-38.9249, 4.3469) (-38.895, 4.3625) (-38.8635, 4.3757) (-38.8305, 4.3845) (-38.797, 4.3907) (-38.7743, 4.3914) (-38.7629, 4.3917) knots 0 0 0 0 0.094687 0.181994 0.264377 0.34218 0.418618 0.496509 0.577369 0.661511 0.746733 0.831258 0.915206 1 1 1 1
  spline S32 degree 3 poles (-38.7629, 4.3917) (-38.7518, 4.3914) (-38.7299, 4.3908) (-38.6976, 4.3862) (-38.6665, 4.379) (-38.6368, 4.3684) (-38.608, 4.3554) (-38.5808, 4.3388) (-38.5545, 4.3197) (-38.5298, 4.2978) (-38.5072, 4.2737) (-38.4872, 4.2479) (-38.4706, 4.2204) (-38.4566, 4.1916) (-38.4459, 4.1612) (-38.4383, 4.1295) (-38.4339, 4.0962) (-38.4333, 4.0735) (-38.433, 4.062) knots 0 0 0 0 0.064207 0.126425 0.18768 0.248216 0.308305 0.369661 0.431699 0.495947 0.559758 0.622295 0.683911 0.745092 0.80674 0.869087 0.93329 1 1 1 1
  spline S33 degree 3 poles (-38.433, 4.062) (-38.4332, 4.0516) (-38.4337, 4.0311) (-38.4376, 4.0013) (-38.4444, 3.973) (-38.4538, 3.9462) (-38.4658, 3.9209) (-38.4805, 3.897) (-38.4981, 3.8748) (-38.5182, 3.8543) (-38.5402, 3.8354) (-38.5645, 3.8193) (-38.5906, 3.8058) (-38.6181, 3.7941) (-38.6478, 3.7857) (-38.6791, 3.7794) (-38.7122, 3.7758) (-38.7349, 3.7753) (-38.7465, 3.775) knots 0 0 0 0 0.065351 0.127916 0.18836 0.247216 0.30563 0.36377 0.422661 0.482687 0.5433 0.604118 0.664965 0.727413 0.791468 0.858055 0.927037 1 1 1 1
  spline S34 degree 3 poles (-38.7465, 3.775) (-38.7566, 3.7752) (-38.7774, 3.7757) (-38.8093, 3.7789) (-38.8428, 3.7842) (-38.8779, 3.7915) (-38.9145, 3.801) (-38.9526, 3.8124) (-38.9924, 3.8261) (-39.0192, 3.8364) (-39.033, 3.8417) knots 0 0 0 0 0.102203 0.211023 0.3251 0.446502 0.573788 0.708901 0.850358 1 1 1 1
  point P0 (47.8, 44)
  point P1 (-27.383, 6.7417)
  constraints: 140 end point, 34 point on circle, 19 centre point, 4 symmetric about line, 74 other
extrude "Выдавливание10" cut sketch "Эскиз11" against normal blind 18 contours A17 | A18
